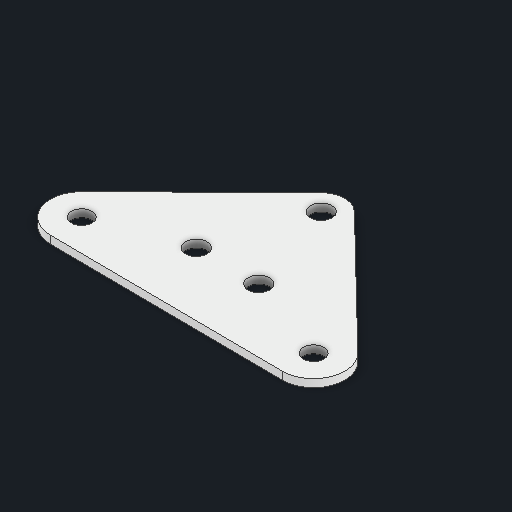
# Autodesk Inventor part: MOGO Clamp Gusset
Saved by Autodesk Inventor 2025.1 (Build 291241000, 241)
## iProperties
Created: 2024-11-26
Part Number: MOGO Clamp Gusset
Material: Acetal Resin, White
Document SubType Name: Sheet Metal
Designer: avere
Density: 1.425 g/cm^3
Appearance: Smooth - White
Flat Pattern Width: 3.65862 cm
Flat Pattern Length: 6.02137 cm
Flat Pattern Area: 22.0299 cm^2
Sheet Metal Rule: Default_mm
Sheet Metal Width: 1.440 in
Sheet Metal Length: 2.371 in
Sheet Metal Area: 3.415 in^2
Author: avere
Autodesk Inventor part; units mm, degrees
ref_plane "YZ Plane" through (0, 0, 0) normal (1, 0, 0) x (0, 1, 0)
ref_plane "XZ Plane" through (0, 0, 0) normal (0, 1, 0) x (-1, 0, 0)
ref_plane "XY Plane" through (0, 0, 0) normal (0, 0, 1) x (1, 0, 0)
sketch "Sketch1" plane through (0, 0, 0) normal (0, 1, 0) x (-1, 0, 0)
  circle A0 centre (5.98, -1.0093) radius 2.1844
  circle A1 centre (-6.72, -1.0093) radius 2.1844
  arc A2 (25.9781, -0.3931) -> (23.0279, 11.58) centre (23.0279, 5.23) ccw
  arc A3 (-24.4341, 11.9556) -> (-27.4345, -0.0172) centre (-24.4843, 5.6058) ccw
  circle A4 centre (23.0279, 5.23) radius 2.0955
  circle A5 centre (-24.4843, 5.6058) radius 2.0955
  line L0 (23.0279, 11.58) -> (-24.4341, 11.9556)
  circle A6 centre (-0.37, -20.0593) radius 2.1844
  arc A7 (-3.6903, -23.4735) -> (2.973, -23.4513) centre (-0.37, -20.0593) ccw
  line L1 (27.4853, 0.7073) -> (2.973, -23.4513)
  line L2 (-28.9114, 1.0535) -> (-3.6903, -23.4735)
  point P0 (0, 0)
  dimension "d0" = 12.7
  dimension "d1" = 12.7
  dimension "d2" = 4.191
  dimension "d3" = 4.191
  dimension "d4" = 9.525
  dimension "d7" = 6.2393
  dimension "d8" = 17.0479
  constraints: 8 centre point, 8 point on circle, 6 end point, 5 tangent, 3 coincident, 3 other
  measures "d0" diameter of A2
  measures "d1" diameter of A3
  measures "d2" diameter of A4
  measures "d3" diameter of A5
  measures "d4" diameter of A7
  measures "d7" vertical distance of A0.centre A2.centre
  measures "d8" horizontal distance of A0.centre A2.centre
extrude "Extrusion1" add sketch "Sketch1" along normal blind 1.5875
equation "\"BendRadius\" = Thickness"
equation "\"BendReliefWidth\" = Thickness"
equation "\"BendReliefDepth\" = 0.5 * Thickness"
equation "\"CornerReliefSize\" = 4 * Thickness"
equation "\"MinimumRemnant\" = 2 * Thickness"
equation "\"TransitionRadius\" = BendRadius"
equation "\"JacobiRadiusSize\" = BendRadius"
equation "\"GapSize\" = Thickness"
equation "\"Thickness\" = 1.5875"
body "Solid1"
